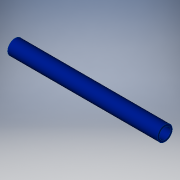
# Autodesk Inventor part: PIJM20-15-200
Saved by Autodesk Inventor 2019 (Build 230136000, 136)
## iProperties
Created: 2022-11-22
Part Number: PIJM20-15-200
Material: Generic
Catalog Web Link: www.cadenas.de
Description: PIJJ, PIJK, PIJM, PIJW, PIJG, PIJT, PIJB, PIJN, PIJF, PIJP, PIJS, PIJX, PIJU-Resin Pipes - ID and OD Surface Finished
Vendor: MISUMI
Document SubType Name: Modeling
Designer: psAdmin
Manufacturer: MISUMI
Mass: 27.4889 g
Surface Area: 222.66 cm^2
Volume: 27.4889 cm^3
Density: 1 g/cm^3
Appearance: PSOLRGB-0-127-255
Category: PARTsolutions
Company: MISUMI
Title: PIJM20-15-200
Author: Cadenas PARTsolutions
Comments: Resin Pipes - ID and OD Surface Finished
PSOL_IDENT_0: {$CADENAS_DATA/23d-libs/misumi/metric/22_rods_pipes/pijj.prj},259 {VTYP=3D},{NB=PIJM20-15-200},{LINA=
PSOL_IDENT_1: PIJM20-15-200},{NN=PIJJ, PIJK, PIJM, PIJW, PIJG, PIJT, PIJB, PIJN, PIJF, PIJP, PIJS, PIJX, PIJU},{DA
PSOL_IDENT_2: TE=30.06.2021 13:08:38},{GEOMDATE=29.05.2014 00:00:00},{VERSION=},{LINEID=120},{WBVAR=MAT,GRADE,COLO
PSOL_IDENT_3: R,V,L},{WBNUMERIC=V,L}  {NB=PIJM20-15-200},{LINA=PIJM20-15-200},{KT=DUMMY},{PN=PIJM20-15-200},{TYPE=
PSOL_IDENT_4: PIJM},{MAT=MC},{MATALG= 'P','Polyacetal','MC','MC Nylon','B','Bakelite','F','Fluororesin','PEEK','PE
PSOL_IDENT_5: EK','PPS','PPS','ABS','ABS Resin','UHMWP','Ultra-High-Molecular-Weight-Polyethylene' },{GRADE=S},{GR
PSOL_IDENT_6: ADEALG= 'S','Standard','CDR2','Conductive CDR2','CDR6','Conductive CDR6' },{COLOR=BL},{COLORALG= 'BL'
PSOL_IDENT_7: ,'Blue','I','Ivory' },{COL=0.00,0.50,1.00,0.00},{D=20},{V=15},{VALG=8,10,12,15},{L=200},{LALG=[20:20
PSOL_IDENT_8: 0/1]},{LMIN=20},{LMAX=200}
NB: PIJM20-15-200
NN: PIJJ, PIJK, PIJM, PIJW, PIJG, PIJT, PIJB, PIJN, PIJF, PIJP, PIJS, PIJX, PIJU
NT: Resin Pipes - ID and OD Surface Finished
NBSYN: $PN.
LINA: PIJM20-15-200
CATALOG: Misumi
PN: PIJM20-15-200
MAT: MC Nylon
GRADE: Standard
COLOR: Blue
D: 20
V: 15
L: 200
SUPPLIER: MISUMI
ARTICLENO: PIJM20-15-200
BOMINFO: PIJM20-15-200
CREATOR: CADENAS GmbH
Autodesk Inventor part; units mm, degrees
ref_plane "YZ Plane" through (0, 0, 0) normal (1, 0, 0) x (0, 1, 0)
ref_plane "XZ Plane" through (0, 0, 0) normal (0, 1, 0) x (-1, 0, 0)
ref_plane "XY Plane" through (0, 0, 0) normal (0, 0, 1) x (1, 0, 0)
sketch "Sketch_1" plane through (0, 0, 0) normal (0, 0, 1) x (1, 0, 0)
  line L0 (200, 0) -> (0, 0)
  line L1 (0, 7.5) -> (200, 7.5)
  line L2 (200, 7.5) -> (200, 10)
  line L3 (200, 10) -> (0, 10)
  line L4 (0, 10) -> (0, 7.5)
  constraints: 10 end point
revolve "Revolution1" add sketch "Sketch_1" angle 360 about axis through (200, 0, 0) along (1, 0, 0)
body "Solid1"
